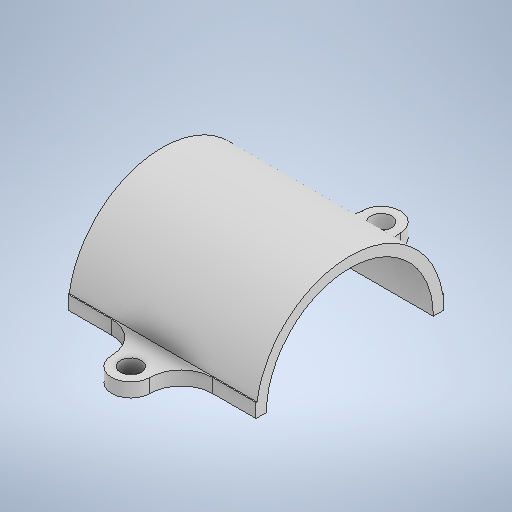
# Autodesk Inventor part: daisen_moto_parts2
Saved by Autodesk Inventor 2025.2 (Build 292293000, 293)
## iProperties
Created: 2025-01-13
Part Number: daisen_moto_parts2
Material: 一般
Document SubType Name: Modeling
Designer: mahhy
Density: 1 g/cm^3
Appearance: 既定
Author: mahhy
Autodesk Inventor part; units mm, degrees
ref_plane "YZ Plane" through (0, 0, 0) normal (1, 0, 0) x (0, 1, 0)
ref_plane "XZ Plane" through (0, 0, 0) normal (0, 1, 0) x (-1, 0, 0)
ref_plane "XY Plane" through (0, 0, 0) normal (0, 0, 1) x (1, 0, 0)
sketch "スケッチ1" plane through (0, 0, 0) normal (0, 1, 0) x (-1, 0, 0)
  line L0 (0, 0) -> (27, 0)
  line L1 (27, 0) -> (27, -27)
  line L2 (27, -27) -> (0, -27)
  line L3 (0, -27) -> (0, 0)
  circle A0 centre (13.5, 4.5) radius 2.75
  line L4 (16.25, 4.5) -> (20.75, 4.5)
  line L5 (10.75, 4.5) -> (6.25, 4.5)
  arc A1 (16.25, 4.5) -> (20.75, 0) centre (20.75, 4.5) ccw
  arc A2 (6.25, 0) -> (10.75, 4.5) centre (6.25, 4.5) ccw
  circle A3 centre (13.5, -31.5) radius 2.75
  line L6 (10.75, -31.5) -> (6.25, -31.5)
  line L7 (16.25, -31.5) -> (20.75, -31.5)
  arc A4 (20.75, -27) -> (16.25, -31.5) centre (20.75, -31.5) ccw
  arc A5 (10.75, -31.5) -> (6.25, -27) centre (6.25, -31.5) ccw
  dimension "d0" = 27
  dimension "d1" = 27
  dimension "d11" = 5.5
  dimension "d12" = 4.5
  dimension "d13" = 4.5
  dimension "d14" = 4.5
  dimension "d15" = 5.5
  dimension "d16" = 4.5
  dimension "d17" = 4.5
  dimension "d18" = 4.5
  constraints: 16 end point, 12 point on circle, 6 centre point, 5 coincident, 5 horizontal, 4 point on line, 2 parallel, 1 perpendicular
  measures "d0" distance of L1.end L3.start
  measures "d1" distance of L0.end L1.end
  measures "d11" diameter of A0
  measures "d12" distance from line of L0 A0.centre
  measures "d13" distance of L4.start L4.end
  measures "d14" distance of L5.start L5.end
  measures "d15" diameter of A3
  measures "d16" distance from line of L2 A3.centre
  measures "d17" distance of L6.start L6.end
  measures "d18" distance of L7.start L7.end
extrude "押し出し1" add sketch "スケッチ1" along normal blind 2
sketch "スケッチ2" plane through (0, 0, 0) normal (1, 0, 0) x (0, 0, -1)
  line L0 (27, 0) -> (0, 0) projected
  circle A0 centre (13.5, 0) radius 13.5
  line L1 (27, 2) -> (0, 2)
  line L2 (0.149, 2) -> (26.851, 2)
  dimension "d21" = 27
  constraints: 4 end point, 2 point on circle, 2 point on line, 1 centre point, 1 midpoint
  measures "d21" diameter of A0
extrude "押し出し2" add sketch "スケッチ2" against normal blind 27 contours L1 A0
sketch "スケッチ3" plane through (0, 2, 0) normal (0, 1, 0) x (1, 0, 0)
  arc A0 (-10.75, 31.5) -> (-16.25, 31.5) centre (-13.5, 31.5) ccw projected
  arc A1 (-16.25, -4.5) -> (-10.75, -4.5) centre (-13.5, -4.5) ccw projected
  point P0 (0, 0)
  constraints: 2 coincident
hole "穴1" at (-13.5, 2, -31.5) at (-13.5, 2, 4.5) direction (0, -1, 0) diameter 3 end through all
sketch "スケッチ4" plane through (0, 0, 0) normal (1, 0, 0) x (0, 0, -1)
  line L0 (27, 0) -> (0, 0) projected
  circle A0 centre (13.5, 0) radius 12
  point P0 (1.5, 0)
  point P1 (25.5, 0)
  dimension "d31" = 24
  constraints: 1 centre point, 1 midpoint
  measures "d31" diameter of A0
extrude "押し出し3" cut sketch "スケッチ4" against normal through all contours L0 A0 picked at (16.494, 4.567)
